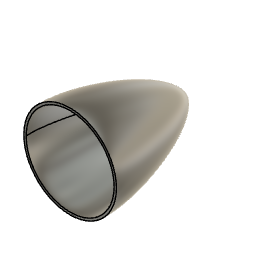
Nose Cones v1 (Autodesk Fusion 360 design; units mm, degrees)
Autodesk Fusion 360 part; units mm, degrees
sketch "Sketch1" plane through (0, 0, 0) normal (0, 0, 1) x (1, 0, 0)
  line L0 (-50.8, 0) -> (0, 0)
  line L1 (0, 0) -> (0, 127)
  line L2 (-50.8, 0) -> (-53.34, 27.94)
  line L3 (-53.34, 27.94) -> (-33.02, 104.14)
  line L4 (-33.02, 104.14) -> (-12.7, 121.92)
  line L5 (-12.7, 121.92) -> (0, 127)
  spline S0 degree 4 poles (-50.8, 0) (-53.34, 27.94) (-33.02, 104.14) (-12.7, 121.92) (0, 127) knots 0 0 0 0 0 1 1 1 1 1
  constraint coincident L0.end L1.start
  constraint horizontal L0
  constraint perpendicular L0 L1
revolve "Revolve1" add sketch "Sketch1" angle 360 about axis through (0, 0, 0) along (0, 1, 0) contours L0 L1 S0
shell "Shell1" thickness 2.54 removed faces 1 at (15.2686, 0, 3.3639)
